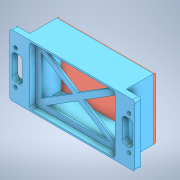
# Autodesk Inventor part: BodyStructure Front
Saved by Autodesk Inventor 2022.2 (Build 262287030, 287C)
## iProperties
Created: 2019-11-06
Part Number: BodyStructure Front
Material: solidworks materials|ABS
Document SubType Name: Modeling
Designer: Jochen
Density: 1.02 g/cm^3
Appearance: 255,255,255
Sending System: SolidWorks 2017
Last Author: Felix
Last Saved: 2021-02-23
Author: Jochen
Autodesk Inventor part; units mm, degrees
ref_plane "YZ Plane" through (0, 0, 0) normal (1, 0, 0) x (0, 1, 0)
ref_plane "XZ Plane" through (0, 0, 0) normal (0, 1, 0) x (-1, 0, 0)
ref_plane "XY Plane" through (0, 0, 0) normal (0, 0, 1) x (1, 0, 0)
sketch "Sketch1" plane through (0, 0, 0) normal (0, 0, 1) x (1, 0, 0)
  line L0 (0, -37.8) -> (0, 37.8) construction
  line L1 (-77, 0) -> (77, 0) construction
  line L2 (-55, -27) -> (55, -27)
  line L3 (55, -27) -> (55, 27)
  line L4 (55, 27) -> (-55, 27)
  line L5 (-55, 27) -> (-55, -27)
  line L6 (-53, -11) -> (-44, -11)
  line L7 (-44, -11) -> (-44, 11)
  line L8 (-44, 11) -> (-53, 11)
  line L9 (-53, 11) -> (-53, -11)
  line L10 (44, -11) -> (53, -11)
  line L11 (53, -11) -> (53, 11)
  line L12 (53, 11) -> (44, 11)
  line L13 (44, 11) -> (44, -11)
  line L14 (-37.5, -25.5) -> (-37.5, 25.5)
  line L15 (37.5, 25.5) -> (37.5, -25.5)
  circle A0 centre (-50, -15) radius 1.5
  circle A1 centre (-50, 15) radius 1.5
  circle A2 centre (50, 15) radius 1.5
  circle A3 centre (50, -15) radius 1.5
  line L16 (-50, -15) -> (50, -15) construction
  line L17 (50, -15) -> (50, 15) construction
  line L18 (50, 15) -> (-50, 15) construction
  line L19 (-50, 15) -> (-50, -15) construction
  line L20 (-55, 0) -> (55, 0) construction
  line L21 (-37.5, 25.5) -> (37.5, 25.5)
  line L22 (-37.5, -25.5) -> (37.5, -25.5)
  line L23 (-42.5, 27) -> (-42.5, -27)
  line L24 (42.5, 27) -> (42.5, -27)
  line L25 (32.5, 17.5442) -> (32.5, -17.5442)
  line L26 (32.5, 17.5442) -> (4.686, 0)
  line L27 (32.5, -17.5442) -> (4.686, 0)
  line L28 (0, 2.9558) -> (-27.814, 20.5)
  line L29 (-27.814, 20.5) -> (27.814, 20.5)
  line L30 (27.814, 20.5) -> (0, 2.9558)
  line L31 (-32.5, 17.5442) -> (-4.686, 0)
  line L32 (-4.686, 0) -> (-32.5, -17.5442)
  line L33 (-32.5, -17.5442) -> (-32.5, 17.5442)
  line L34 (0, -2.9558) -> (-27.814, -20.5)
  line L35 (-27.814, -20.5) -> (27.814, -20.5)
  line L36 (27.814, -20.5) -> (0, -2.9558)
  point P0 (0, 0)
  dimension "d0" = 22
  dimension "d1" = 3
  dimension "d2" = 9
  dimension "d3" = 54
  dimension "d4" = 110
  dimension "d5" = 2
  dimension "d6" = 75
  dimension "d7" = 100
  dimension "d8" = 30
  dimension "d14" = 51
  dimension "d15" = 85
  dimension "d44" = 5
  dimension "d45" = 5
  dimension "d46" = 5
  constraints: 70 end point, 14 parallel, 9 point on line, 7 horizontal, 6 perpendicular, 5 collinear, 4 centre point, 4 equal length, 3 equal radius, 3 midpoint, 2 coincident, 2 vertical, 18 other
  measures "d0" distance of L10.end L11.end
  measures "d1" diameter of A3
  measures "d2" distance between parallel lines of L11 L13
  measures "d3" distance of L2.end L3.end
  measures "d4" distance of L3.end L4.end
  measures "d5" distance from line of L20.end L11
  measures "d6" distance between parallel lines of L15 L14
  measures "d7" distance of L17.end L18.end
  measures "d8" distance of L18.end L16.start
  measures "d14" distance of L14.start L14.end
  measures "d15" distance between parallel lines of L24 L23
  measures "d44" distance between parallel lines of L29 L21
  measures "d45" distance between parallel lines of L25 L15
  measures "d46" distance between parallel lines of L26 L30
extrude "Extrusion1" add sketch "Sketch1" against normal blind 10 contours L5 L4 L23 L2 | L23 L4 L24 L2 | L24 L4 L3 L2 | L14 L21 L15 L22
extrude "Extrusion2" cut sketch "Sketch1" along normal blind 3.5 from surface at -10 contours L14 L21 L15 L22 | L25 L27 L26 | L28 L29 L30 | L31 L32 L33 | L36 L35 L34
extrude "Extrusion10" cut sketch "Sketch1" against normal blind 5 contours L14 L21 L15 L22
extrude "Extrusion3" cut sketch "Sketch1" along normal blind 5 from surface at -10 contours L5 L4 L23 L2 | L24 L4 L3 L2
fillet "Fillet1" radius 2 8 edges at (55, 27, -2.5) (55, -27, -2.5) (-55, 27, -2.5) (-55, -27, -2.5) (-37.5, 25.5, -2.5) (-37.5, -25.5, -2.5) (37.5, 25.5, -2.5) (37.5, -25.5, -2.5)
fillet "Fillet2" radius 3 8 edges at (-44, -11, -2.5) (-53, -11, -2.5) (44, -11, -2.5) (53, -11, -2.5) (53, 11, -2.5) (44, 11, -2.5) (-53, 11, -2.5) (-44, 11, -2.5)
sketch "Sketch2" plane through (0, 0, -10) normal (0, 0, -1) x (-1, 0, 0)
  line L0 (37.5, 25.5) -> (-37.5, 25.5)
  line L1 (-37.5, 25.5) -> (-37.5, -25.5)
  line L2 (-37.5, -25.5) -> (37.5, -25.5)
  line L3 (37.5, -25.5) -> (37.5, 25.5)
  line L4 (-42.5, 27) -> (-42.5, -27) projected
  line L5 (-42.5, -27) -> (42.5, -27) projected
  line L6 (42.5, -27) -> (42.5, 27) projected
  line L7 (42.5, 27) -> (-42.5, 27) projected
  line L8 (0, -38.3799) -> (0, 38.3799) construction
  line L9 (77.5799, 0) -> (-77.5799, 0) construction
  line L10 (42.5, 27) -> (42.5, -27) projected
  line L11 (42.5, 27) -> (53, 27)
  line L12 (55, 25) -> (55, -25)
  line L13 (55, 25) -> (55, -25) projected
  line L14 (42.5, -27) -> (53, -27)
  line L15 (-42.5, -27) -> (-42.5, 27) projected
  line L16 (-42.5, 27) -> (-53, 27)
  line L17 (-55, 25) -> (-55, -25)
  line L18 (-55, -25) -> (-55, 25) projected
  line L19 (-42.5, -27) -> (-53, -27)
  line L20 (-44, -8) -> (-44, 8) projected
  circle A0 centre (44.5, 0) radius 1.15
  circle A1 centre (-44.5, 0) radius 1.15
  arc A2 (55, 25) -> (53, 27) centre (53, 25) ccw
  arc A3 (53, -27) -> (55, -25) centre (53, -25) ccw
  arc A4 (-53, 27) -> (-55, 25) centre (-53, 25) ccw
  arc A5 (-55, -25) -> (-53, -27) centre (-53, -25) ccw
  circle A6 centre (-50, 15) radius 1.5 projected
  circle A7 centre (-50, -15) radius 1.5 projected
  circle A8 centre (50, -15) radius 1.5 projected
  circle A9 centre (50, 15) radius 1.5 projected
  circle A10 centre (-50, 15) radius 3
  circle A11 centre (-50, -15) radius 3
  circle A12 centre (50, -15) radius 3
  circle A13 centre (50, 15) radius 3
  point P0 (0, 0)
  point P1 (55, 27)
  point P2 (55, -27)
  point P3 (-55, 27)
  point P4 (-55, -27)
  point P5 (47.75, -27)
  point P6 (47.75, 27)
  dimension "d24" = 54
  dimension "d26" = 2.3
  dimension "d27" = 2
  dimension "d36" = 2
  dimension "d43" = 6
  constraints: 20 end point, 18 point on line, 10 centre point, 8 point on circle, 8 tangent, 7 equal radius, 5 coincident, 3 horizontal, 3 perpendicular, 2 collinear, 2 midpoint, 2 parallel, 4 other
  measures "d24" distance of point (47.75, -27) point (47.75, 27)
  measures "d26" diameter of A0
  measures "d27" distance from line of L6 A0.centre
  measures "d36" radius of A2
  measures "d43" diameter of A10
extrude "Extrusion4" add sketch "Sketch2" along normal blind 19 contours L7 L6 L5 L4
sketch "Sketch3" plane through (0, 0, -29) normal (0, 0, -1) x (-1, 0, 0)
  line L0 (37.5, -25.5) -> (37.5, 25.5) projected
  line L1 (37.5, 25.5) -> (-37.5, 25.5) projected
  line L2 (-37.5, 25.5) -> (-37.5, -25.5) projected
  line L3 (-37.5, -25.5) -> (37.5, -25.5) projected
  line L4 (37.3, 25.3) -> (37.3, -25.3)
  line L5 (37.3, -25.3) -> (-37.3, -25.3)
  line L6 (-37.3, -25.3) -> (-37.3, 25.3)
  line L7 (-37.3, 25.3) -> (37.3, 25.3)
  line L8 (42.5, -27) -> (-42.5, -27) projected
  line L9 (-42.5, -27) -> (-42.5, 27) projected
  line L10 (-37.5, -25.5) -> (37.5, -25.5) projected
  line L11 (37.5, -25.5) -> (37.5, 25.5) projected
  line L12 (37.5, 25.5) -> (-37.5, 25.5) projected
  line L13 (-37.5, 25.5) -> (-37.5, -25.5) projected
  line L14 (42.5, -27) -> (-42.5, -27) projected
  line L15 (-42.5, -27) -> (-42.5, 27) projected
  line L16 (0, -37.8) -> (0, 37.8) construction
  circle A0 centre (-40, 0) radius 1.15
  circle A1 centre (40, 0) radius 1.15
  line L17 (-42.5, -27) -> (-42.5, 27) projected
  line L18 (-42.5, 0) -> (-37.5, 0) construction
  line L19 (-42.5, 27) -> (42.5, 27) projected
  line L20 (-42.5, 27) -> (42.5, 27) projected
  line L21 (42.5, 27) -> (42.5, -27) projected
  line L22 (42.5, 27) -> (42.5, -27) projected
  point P0 (0, 0)
  point P1 (-45, 15)
  point P2 (-45, -15)
  point P3 (45, -15)
  point P4 (45, 15)
  dimension "d31" = 0.2
  dimension "d48" = 2.3
  constraints: 10 end point, 4 midpoint, 2 centre point, 4 other
  measures "d31" distance between parallel lines of L0 L4
  measures "d48" diameter of A0
extrude "Extrusion8" cut sketch "Sketch3" against normal blind 5 contours A0 | A1
extrude "Extrusion9" add sketch "Sketch3" along normal blind 2 separate body contours L3 L2 L1 L0 | L4 L5 L6 L7 | L8 L9 L19 L21
extrude "Extrusion7" add sketch "Sketch3" against normal blind 1 contours L4 L5 L6 L7 bodies 2
fillet "Fillet5" radius 2 2 edges at (0, 27, -31) (0, -27, -31)
body "Solid1"
